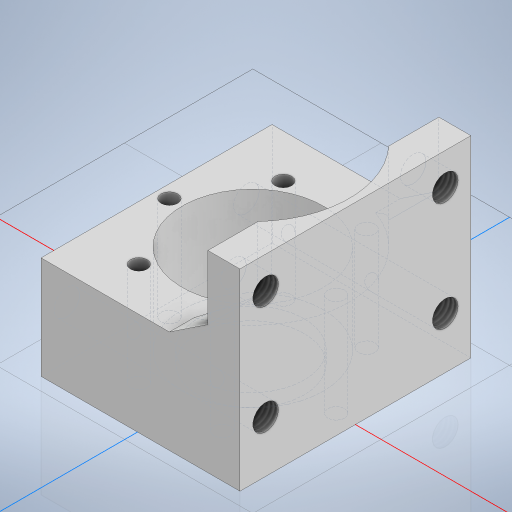
# Autodesk Inventor part: OsBase
Saved by Autodesk Inventor 2024 (Build 280153000, 153)
## iProperties
Created: 2023-08-20
Part Number: OsBase
Material: Generic
Document SubType Name: Modeling
Designer: KirikDK
Density: 1 g/cm^3
Appearance: Default
Author: KirikDK
Autodesk Inventor part; units mm, degrees
ref_plane "YZ Plane" through (0, 0, 0) normal (1, 0, 0) x (0, 1, 0)
ref_plane "XZ Plane" through (0, 0, 0) normal (0, 1, 0) x (-1, 0, 0)
ref_plane "XY Plane" through (0, 0, 0) normal (0, 0, 1) x (1, 0, 0)
sketch "Sketch1" plane through (0, 0, 0) normal (0, 1, 0) x (-1, 0, 0)
  circle A0 centre (0, 0) radius 11
  line L0 (15, 18) -> (-16, 18)
  line L1 (-16, 18) -> (-16, -18)
  line L2 (-16, -18) -> (15, -18)
  line L3 (15, -18) -> (15, 18)
  dimension "d0" = 22
  dimension "d1" = 15
  dimension "d2" = 16
  dimension "d3" = 18
  dimension "d4" = 18
  constraints: 8 end point, 2 parallel, 1 centre point, 1 coincident, 1 horizontal, 1 perpendicular
  measures "d0" diameter of A0
  measures "d1" distance from line of point (0, 0) L3
  measures "d2" distance from line of L1 point (0, 0)
  measures "d3" distance from line of L0 point (0, 0)
  measures "d4" distance from line of point (0, 0) L2
extrude "Extrusion1" add sketch "Sketch1" along normal blind 30
sketch "Sketch3" plane through (16, 0, -18) normal (0, 0, -1) x (-1, 0, 0)
  line L0 (5, 30) -> (5, 0) projected
  line L1 (5, 30) -> (5, 20)
  line L2 (5, 20) -> (11, 16)
  line L3 (11, 16) -> (31, 16)
  line L4 (31, 16) -> (31, 0)
  line L5 (31, 0) -> (1, 0)
  line L6 (1, 0) -> (1, 30)
  line L7 (1, 30) -> (5, 30)
  line L8 (31, 0) -> (31, 30) projected
  line L9 (31, 16) -> (31, 30)
  line L10 (31, 30) -> (5, 30)
  line L11 (5, 30) -> (5, 20)
  line L12 (5, 20) -> (11, 16)
  line L13 (11, 16) -> (31, 16)
  point P0 (16, 0)
  dimension "d7" = 16
  constraints: 24 end point, 4 perpendicular, 2 collinear, 2 point on line, 2 vertical
  measures "d7" distance of L3.end L4.end
extrude "Extrusion2" cut sketch "Sketch3" against normal up to surface (36 mm away) contours L10 L8 L3 L2 L0
sketch "Sketch4" plane through (0, 30, 0) normal (0, 1, 0) x (1, 0, 0)
  circle A0 centre (0, 0) radius 15
  dimension "d24" = 30
  constraints: 1 centre point, 1 coincident
  measures "d24" diameter of A0
extrude "Extrusion3" cut sketch "Sketch4" against normal blind 14
sketch "Sketch5" plane through (0, 0, 0) normal (0, -1, 0) x (1, 0, 0)
  circle A0 centre (0, 0) radius 11
  circle A1 centre (-0.289, 0) radius 8.289
  constraints: 2 centre point, 1 coincident
extrude "Extrusion4" add sketch "Sketch5" against normal blind 2
sketch "Sketch6" plane through (11, 20, 18) normal (-1, 0, 0) x (0, 0, 1)
  circle A0 centre (-4, -12) radius 2
  circle A1 centre (-32, -12) radius 2
  circle A2 centre (-32, 5) radius 2
  circle A3 centre (-4, 5) radius 2
  point P0 (-18, -20)
  constraints: 4 centre point
extrude "Extrusion5" cut sketch "Sketch6" along normal mid plane 200
thread "Thread1" size "M4x0.7" class "6H" standard "ANSI Metric M Profile" full length
thread "Thread2" size "M4x0.7" class "6H" standard "ANSI Metric M Profile" full length
thread "Thread3" size "M4x0.7" class "6H" standard "ANSI Metric M Profile" full length
thread "Thread4" size "M4x0.7" class "6H" standard "ANSI Metric M Profile" full length
sketch "Sketch7" plane through (-15, 16, -18) normal (0, 1, 0) x (1, 0, 0)
  arc A0 (26, -7.802) -> (20, -3.8579) centre (15, -18) ccw projected
  circle A1 centre (15, -18) radius 15
  circle A2 centre (28, -18) radius 1.3
  circle A3 centre (21.5, -6.7417) radius 1.3
  circle A4 centre (8.5, -6.7417) radius 1.3
  circle A5 centre (2, -18) radius 1.3
  circle A6 centre (8.5, -29.2583) radius 1.3
  circle A7 centre (21.5, -29.2583) radius 1.3
  point P0 (15, -18)
  dimension "d25" = 2.6
  dimension "d26" = 13
  dimension "d29" = 360
  constraints: 6 centre point, 1 coincident, 16 other
  measures "d25" diameter of A2
  measures "d26" distance of A2.centre point (15, -18)
extrude "Extrusion6" cut sketch "Sketch7" against normal blind 200 contours A2 | A3 | A4 | A5 | A6 | A7
body "Solid1"
